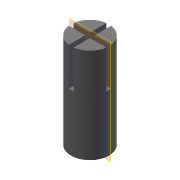
# Autodesk Inventor part: workfeatures2
Saved by Autodesk Inventor 2022 Beta2 (Build 260130000, 130) ContinuousBuild 0
## iProperties
Created: 2008-03-12
Part Number: workfeatures2
Document SubType Name: Modeling
Designer: jmacmillan
Density: 1 g/cm^3
Mass: 226.767 g
Surface Area: 319.795 cm^2
Volume: 226.767 cm^3
Material: Generic
Appearance: Light Gray
Author: jmacmillan
Autodesk Inventor part; units mm, degrees
ref_plane "YZ Plane" through (0, 0, 0) normal (1, 0, 0) x (0, 1, 0)
ref_plane "XZ Plane" through (0, 0, 0) normal (0, 1, 0) x (-1, 0, 0)
sketch "Sketch1" plane through (0, 0, 0) normal (0, 1, 0) x (-1, 0, 0)
  circle A0 centre (0, 0) radius 25.4
  dimension "d1" = 50.8
  constraints: 1 centre point, 1 coincident
  measures "d1" diameter of A0
extrude "Extrusion1" add sketch "Sketch1" along normal blind 127
sketch "Sketch2" plane through (0, 127, 0) normal (0, 1, 0) x (1, 0, 0)
  line L0 (-3.175, -25.2008) -> (-3.175, -3.175)
  line L1 (-3.175, 3.175) -> (-3.175, 25.2008)
  line L2 (25.2008, 3.175) -> (3.175, 3.175)
  line L3 (-3.175, 3.175) -> (-25.2008, 3.175)
  line L4 (3.175, 25.2008) -> (3.175, 3.175)
  line L5 (3.175, -3.175) -> (3.175, -25.2008)
  line L6 (-25.2008, -3.175) -> (-3.175, -3.175)
  line L7 (3.175, -3.175) -> (25.2008, -3.175)
  circle A0 centre (0, 0) radius 25.4 construction
  line L8 (0, 35.56) -> (0, -35.56) construction
  line L9 (35.56, 0) -> (-35.56, 0) construction
  arc A1 (3.175, 25.2008) -> (-3.175, 25.2008) centre (0, 0) ccw
  arc A2 (25.2008, -3.175) -> (25.2008, 3.175) centre (0, 0) ccw
  arc A3 (-25.2008, 3.175) -> (-25.2008, -3.175) centre (0, 0) ccw
  arc A4 (-3.175, -25.2008) -> (3.175, -25.2008) centre (0, 0) ccw
  dimension "d11" = 6.35
  dimension "d12" = 6.35
  constraints: 16 end point, 13 point on circle, 8 parallel, 4 centre point, 2 horizontal, 2 horizontal alignment, 2 vertical alignment, 1 concentric, 2 other
  measures "d11" distance between parallel lines of L4 L1
  measures "d12" distance between parallel lines of L3 L6
extrude "Extrusion2" cut sketch "Sketch2" against normal blind 50.8
equation "\"d12\" = d11"
body "Solid1"
